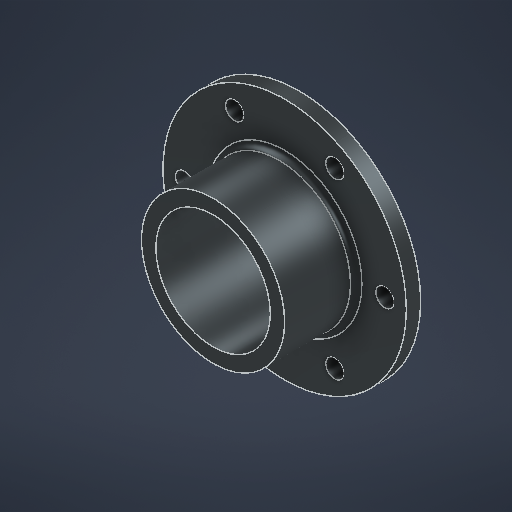
# Autodesk Inventor part: HOSE-NOZZLE-MOUNTING
Saved by Autodesk Inventor 2025.3 (Build 293356030, 356C)
## iProperties
Created: 2025-08-31
Part Number: HOSE-NOZZLE-MOUNTING
Material: Generic
Document SubType Name: Modeling
Designer: lstk1ng
Density: 1 g/cm^3
Appearance: Iron Gray
Author: lstk1ng
Autodesk Inventor part; units mm, degrees
ref_plane "YZ Plane" through (0, 0, 0) normal (1, 0, 0) x (0, 1, 0)
ref_plane "XZ Plane" through (0, 0, 0) normal (0, 1, 0) x (-1, 0, 0)
ref_plane "XY Plane" through (0, 0, 0) normal (0, 0, 1) x (1, 0, 0)
sketch "Sketch7" plane through (0, 0, 0) normal (0, 0, 1) x (1, 0, 0)
  circle A0 centre (0, 0) radius 42.5
  circle A1 centre (0, 0) radius 20
  dimension "d59" = 85
  dimension "d60" = 40
  constraints: 2 centre point, 1 coincident
  measures "d59" diameter of A0
  measures "d60" diameter of A1
extrude "Extrusion6" add sketch "Sketch7" along normal blind 5
sketch "Sketch8" plane through (0, 0, 5) normal (0, 0, 1) x (1, 0, 0)
  circle A0 centre (0, 0) radius 25
  circle A1 centre (0, 0) radius 20 projected
  dimension "d55" = 50
  constraints: 1 centre point, 1 coincident
  measures "d55" diameter of A0
extrude "Extrusion7" add sketch "Sketch8" along normal blind 25
fillet "Fillet4" radius 2 1 edges at (-25, 0, 5)
sketch "Sketch9" plane through (0, 0, 5) normal (0, 0, 1) x (1, 0, 0)
  circle A0 centre (0, 0) radius 35 construction
  circle A1 centre (-35, 0) radius 3.15
  circle A2 centre (-17.5, -30.3109) radius 3.15
  circle A3 centre (17.5, -30.3109) radius 3.15
  circle A4 centre (35, 0) radius 3.15
  circle A5 centre (17.5, 30.3109) radius 3.15
  circle A6 centre (-17.5, 30.3109) radius 3.15
  dimension "d61" = 70
  dimension "d62" = 6.3
  dimension "d65" = 360
  constraints: 6 centre point, 1 coincident, 1 horizontal alignment, 15 other
  measures "d62" diameter of A1
extrude "Extrusion8" cut sketch "Sketch9" against normal through all
body "Solid3"
